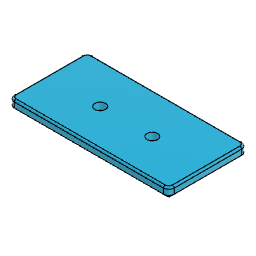
couvercle_connecteur_ILS_KOSMOS3-0 (Autodesk Fusion 360 design; units mm, degrees)
Autodesk Fusion 360 part; units mm, degrees
sketch "Esquisse1" plane through (0, 0, 0) normal (0, 0, 1) x (1, 0, 0)
  line L0 (0, 0) -> (45, 0)
  line L1 (45, 0) -> (45, 22)
  line L2 (45, 22) -> (0, 22)
  line L3 (0, 22) -> (0, 0)
  dimension "d1" = 45
  dimension "d2" = 22
  constraint horizontal L0
  constraint vertical L1
  constraint horizontal L2
  constraint vertical L3
  constraint coincident L0.start L3.end
  measures "d1" distance of L0.start L0.end
  measures "d2" distance of L0.start L2.end
extrude "Extrusion1" add sketch "Esquisse1" along normal blind 2
sketch "Esquisse2" plane through (0, 0, 0) normal (0, 0, -1) x (1, 0, 0)
  line L0 (0, 0) -> (0, -22)
  line L1 (0, -22) -> (45, -22)
  line L2 (45, -22) -> (45, 0)
  line L3 (45, 0) -> (0, 0)
  line L4 (1.4, -20.6) -> (43.6, -20.6)
  line L5 (43.6, -20.6) -> (43.6, -1.4)
  line L6 (43.6, -1.4) -> (1.4, -1.4)
  line L7 (1.4, -1.4) -> (1.4, -20.6)
  dimension "d5" = -1.4
extrude "Extrusion2" add sketch "Esquisse2" along normal blind 1.7 contours L4 L5 L6 L7
fillet "Congé1" radius 1.5 4 edges at (0, 0, 1) (45, 0, 1) (45, 22, 1) (0, 22, 1)
chamfer "Chanfrein1" distance 0.3 angle 45 4 edges at (22.5, 20.6, -1.7) (1.4, 11, -1.7) (22.5, 1.4, -1.7) (43.6, 11, -1.7)
fillet "Congé2" radius 0.5 8 edges at (0.4393, 21.5607, 2) (0, 11, 2) (0.4393, 0.4393, 2) (22.5, 0, 2) (44.5607, 0.4393, 2) (45, 11, 2) (44.5607, 21.5607, 2) (22.5, 22, 2)
hole "Perçage1" at (15.166, 10.5, 2) direction (0, 0, -1) diameter 1.5 depth 9 tip angle 180 counterbore diameter 3 counterbore depth 2
pattern_linear "Réseau R1" count 2 spacing 14.666 along (1, 0, 0) of "Perçage1"
